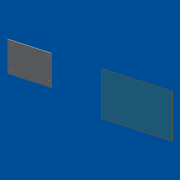
# Autodesk Inventor part: SpartanLap
Saved by Autodesk Inventor 2015 SP1 (Build 190203100, 203)
## iProperties
Created: 2015-04-08
Part Number: SpartanLap
Material: Generic
Document SubType Name: Modeling
Designer: laca
Density: 1 g/cm^3
Appearance: Default
Author: laca
Autodesk Inventor part; units mm, degrees
ref_plane "YZ Plane" through (0, 0, 0) normal (1, 0, 0) x (0, 1, 0)
ref_plane "XZ Plane" through (0, 0, 0) normal (0, 1, 0) x (-1, 0, 0)
ref_plane "XY Plane" through (0, 0, 0) normal (0, 0, 1) x (1, 0, 0)
ref_plane "Work Plane1" through (208.4454, -9.6874, 112.9362) normal (0.2714244, 0, 0.9624598) x (0.9624598, 0, -0.2714244)
sketch "Sketch1" plane through (208.4454, -9.6874, 112.9362) normal (0.2714244, 0, 0.9624598) x (0.9624598, 0, -0.2714244)
  line L0 (-398.5087, 80.1361) -> (-262.5087, 80.1361)
  line L1 (-262.5087, 80.1361) -> (-262.5087, -32.8639)
  line L2 (-262.5087, -32.8639) -> (-398.5087, -32.8639)
  line L3 (-398.5087, -32.8639) -> (-398.5087, 80.1361)
  circle A0 centre (-388.5087, 72.1361) radius 2
  circle A1 centre (-272.5087, 70.1361) radius 2
  circle A2 centre (-298.5087, -22.8639) radius 2
  circle A3 centre (-388.5087, -20.8639) radius 2
  line L4 (-383.5087, -10.8639) -> (-269.5087, -10.8639)
  line L5 (-269.5087, -10.8639) -> (-269.5087, 65.1361)
  line L6 (-269.5087, 65.1361) -> (-383.5087, 65.1361)
  line L7 (-383.5087, 65.1361) -> (-383.5087, -10.8639)
  circle A4 centre (-383.5087, -10.8639) radius 2
  circle A5 centre (-269.5087, -10.8639) radius 2
  circle A6 centre (-269.5087, 65.1361) radius 2
  circle A7 centre (-383.5087, 65.1361) radius 2
  point P0 (-169.9666, 9.6874)
  dimension "d0" = 136
  dimension "d1" = 113
  dimension "d2" = 4
  dimension "d3" = 4
  dimension "d4" = 4
  dimension "d5" = 4
  dimension "d6" = 116
  dimension "d7" = 93
  dimension "d8" = 93
  dimension "d9" = 90
  dimension "d10" = 10
  dimension "d11" = 10
  dimension "d12" = 0
  dimension "d13" = 114
  dimension "d14" = 76
  dimension "d15" = 15
  dimension "d16" = 15
  dimension "d17" = 4
  dimension "d18" = 4
  dimension "d19" = 4
  dimension "d20" = 4
  constraints: 16 end point, 8 centre point, 4 coincident, 4 parallel, 2 horizontal, 2 perpendicular
  measures "d0" distance of L0.start L0.end
  measures "d1" distance of L0.end L1.end
  measures "d2" diameter of A0
  measures "d3" diameter of A1
  measures "d4" diameter of A2
  measures "d5" diameter of A3
  measures "d6" horizontal distance of A1.centre A0.centre
  measures "d7" vertical distance of A2.centre A1.centre
  measures "d8" distance of A3.centre A0.centre
  measures "d9" horizontal distance of A2.centre A3.centre
  measures "d10" distance from line of L2 A2.centre
  measures "d11" distance from line of L3 A3.centre
  measures "d12" horizontal distance of A0.centre A3.centre
  measures "d13" distance of L5.end L6.end
  measures "d14" distance of L6.end L4.start
  measures "d15" distance between parallel lines of L0 L6
  measures "d16" distance between parallel lines of L3 L7
  measures "d17" diameter of A4
  measures "d18" diameter of A5
  measures "d19" diameter of A7
  measures "d20" diameter of A6
extrude "Extrusion1" add sketch "Sketch1" along normal blind 3 contours L0 L1 L2 L3 | L7 A4 L4 | A4 L7 A7 L6 A6 L5 A5 L4 | A5 L5 L4 | L7 L6 A7 | A6 L6 L5 picked at (-383.0711, -9.6133) picked at (-269.9463, -9.6133) picked at (-383.0711, 63.8855) picked at (-269.9463, 63.8855)
extrude "Extrusion2" cut sketch "Sketch1" along normal through all contours L7 A4 L4 | L4 A4 L7 | A5 L5 L4 | L4 L5 A5 | A7 L6 L7 | L7 L6 A7 | A6 L6 L5 | L5 L6 A6
equation "\"d3\" = d2"
equation "\"d4\" = d2"
equation "\"d5\" = d4"
equation "\"d17\" = d4"
equation "\"d18\" = d4"
equation "\"d19\" = d17"
equation "\"d20\" = d18"
body "Solid1"
